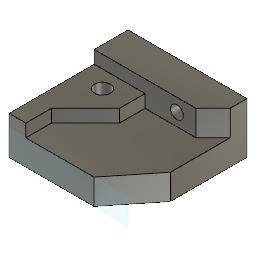
Task1 3C 1 v1 (Autodesk Fusion 360 design; units mm, degrees)
Autodesk Fusion 360 part; units mm, degrees
sketch "Sketch1" plane through (0, 0, 0) normal (0, 0, 1) x (1, 0, 0) in component "box"
  line L0 (70, 70) -> (-70, 70)
  line L1 (-70, 70) -> (-70, -70)
  line L2 (-70, -70) -> (70, -70)
  line L3 (70, -70) -> (70, 70)
  line L4 (70, 70) -> (-70, -70) construction
  line L5 (-70, 70) -> (70, -70) construction
  dimension "d1" = 140
  constraint horizontal L0
  constraint perpendicular L0 L1
  constraint parallel L0 L2
  constraint parallel L1 L3
  constraint coincident L4 origin
  constraint coincident L5 origin
  measures "d1" distance of L1.end L2.end
extrude "Extrude1" add sketch "Sketch1" along normal blind 30 in component "box"
sketch "Sketch2" plane through (0, -70, 0) normal (0, -1, 0) x (1, 0, 0) in component "box"
  line L0 (-70, 0) -> (70, 0)
  line L1 (70, 0) -> (70, 30)
  line L2 (70, 30) -> (-70, 30)
  line L3 (-70, 30) -> (-70, 0)
sketch "Sketch3" plane through (0, 0, 30) normal (0, 0, 1) x (-1, 0, 0) in component "box"
  line L0 (-70, 70) -> (-70, -70)
  line L1 (-70, -70) -> (70, -70)
  line L2 (70, -70) -> (70, 70)
  line L3 (70, 70) -> (-70, 70)
  line L4 (-70, 20) -> (-30, 70)
  line L5 (-30, 70) -> (-70, 70)
  line L6 (-70, 20) -> (-70, 70)
  constraint coincident L0 L4.start
  constraint coincident L3 L4.end
  constraint coincident L0.start L3.end
extrude "Extrude2" cut sketch "Sketch3" against normal up to surface (30 mm away) contours L0 L3 L4 L5 L6 in component "box"
sketch "Sketch4" plane through (0, 0, 30) normal (0, 0, 1) x (-1, 0, 0) in component "box"
  line L0 (-30, 70) -> (-70, 20)
  line L1 (-70, 20) -> (-70, -70)
  line L2 (-70, -70) -> (70, -70)
  line L3 (70, -70) -> (70, 70)
  line L4 (70, 70) -> (-30, 70)
  line L5 (-70, -30) -> (70, -30)
  line L6 (70, -30) -> (70, -70)
  line L7 (70, -70) -> (-70, -70)
  line L8 (-70, -70) -> (-70, -30)
  line L9 (-70, -30) -> (70, -70) construction
  line L10 (70, -30) -> (-70, -70) construction
  point P0 (0, -50)
  constraint horizontal L5
  constraint perpendicular L5 L6
  constraint parallel L5 L7
  constraint parallel L6 L8
  constraint coincident L9 P0
  constraint coincident L10 P0
extrude "Extrude3" add sketch "Sketch4" along normal blind 30 contours L1 L2 L3 L5 L6 L7 L8 in component "box"
sketch "Sketch5" plane through (0, 0, 30) normal (0, 0, 1) x (-1, 0, 0) in component "box"
  line L0 (-70, -30) -> (70, -30)
  line L1 (70, -30) -> (70, 70)
  line L2 (70, 70) -> (-30, 70)
  line L3 (-30, 70) -> (-70, 20)
  line L4 (-70, 20) -> (-70, -30)
  line L5 (10, -30) -> (70, -30)
  line L6 (70, -30) -> (70, 70)
  line L7 (70, 70) -> (10, 70)
  line L8 (10, 70) -> (10, -30)
  line L9 (10, -30) -> (70, 70) construction
  line L10 (70, -30) -> (10, 70) construction
  point P0 (40, 20)
  constraint horizontal L5
  constraint perpendicular L5 L6
  constraint parallel L5 L7
  constraint parallel L6 L8
  constraint coincident L9 P0
  constraint coincident L10 P0
  constraint coincident L0 L5.start
extrude "Extrude4" add sketch "Sketch5" along normal blind 15 contours L0 L1 L2 L5 L6 L7 L8 in component "box"
sketch "Sketch6" plane through (0, 0, 45) normal (0, 0, 1) x (-1, 0, 0) in component "box"
  line L0 (10, 70) -> (10, -30)
  line L1 (10, -30) -> (70, -30)
  line L2 (70, -30) -> (70, 70)
  line L3 (70, 70) -> (10, 70)
  line L4 (50, 70) -> (50, 40)
  line L5 (50, 40) -> (10, 0)
  line L6 (10, 70) -> (50, 70)
  constraint coincident L3 L4.start
  constraint perpendicular L3 L4
  constraint coincident L0 L5.end
  constraint coincident L0.start L3.end
extrude "Extrude5" cut sketch "Sketch6" against normal blind 15 contours L0 L3 L4 L5 L6 in component "box"
sketch "Sketch7" plane through (0, 0, 60) normal (0, 0, 1) x (-1, 0, 0) in component "box"
  line L0 (-70, -70) -> (70, -70)
  line L1 (70, -70) -> (70, -30)
  line L2 (70, -30) -> (-70, -30)
  line L3 (-70, -30) -> (-70, -70)
  line L4 (-70, -50) -> (-50, -30)
  line L5 (-70, -30) -> (-70, -50)
  constraint midpoint L3 L4.start
  constraint coincident L2 L4.end
  constraint coincident L2.end L3.start
extrude "Extrude6" cut sketch "Sketch7" against normal blind 30 contours L2 L3 L4 L5 in component "box"
sketch "Sketch8" plane through (0, 0, 45) normal (0, 0, 1) x (-1, 0, 0) in component "box"
  line L0 (50, 40) -> (10, 0)
  line L1 (10, 0) -> (10, -30)
  line L2 (10, -30) -> (70, -30)
  line L3 (70, -30) -> (70, 70)
  line L4 (70, 70) -> (50, 70)
  line L5 (50, 70) -> (50, 40)
  circle A0 centre (40, -10) radius 9.3121
extrude "Extrude7" cut sketch "Sketch8" against normal blind 45 contours A0 in component "box"
sketch "Sketch9" plane through (0, 30, 0) normal (0, -1, 0) x (1, 0, 0) in component "box"
  line L0 (50, 30) -> (50, 60)
  line L1 (50, 60) -> (-70, 60)
  line L2 (-70, 60) -> (-70, 45)
  line L3 (-70, 45) -> (-10, 45)
  line L4 (-10, 45) -> (-10, 30)
  line L5 (-10, 30) -> (50, 30)
  circle A0 centre (27.54, 44.8379) radius 7.5144
extrude "Extrude8" cut sketch "Sketch9" against normal blind 40 contours A0 in component "box"
component "box" placed x (1, 0, 0) y (0, 1, 0) z (0, 0, 1) at (0, 0, 0)
